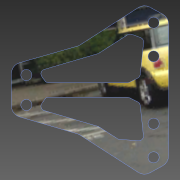
# Autodesk Inventor part: ShoulderBracket
Saved by Autodesk Inventor 2020 (Build 240168000, 168)
## iProperties
Created: 2020-04-01
Part Number: ShoulderBracket
Material: Aluminum 6061
Document SubType Name: Modeling
Designer: valer
Density: 2.7 g/cm^3
Appearance: Aluminum - Flat
Author: valer
Autodesk Inventor part; units mm, degrees
ref_plane "YZ Plane" through (0, 0, 0) normal (1, 0, 0) x (0, 1, 0)
ref_plane "XZ Plane" through (0, 0, 0) normal (0, 1, 0) x (-1, 0, 0)
ref_plane "XY Plane" through (0, 0, 0) normal (0, 0, 1) x (1, 0, 0)
sketch "Base" plane through (0, 0, 0) normal (0, 0, 1) x (1, 0, 0)
  line L0 (0, 0) -> (-82.3214, 0) construction
  line L1 (0, 0) -> (0, -41.0722)
  line L2 (-50.837, -25.008) -> (-13.8922, -48.6905)
  line L3 (-13.8922, -48.6905) -> (0, -41.0722)
  line L4 (-28.3819, -27.8847) -> (-13.9014, -28.9375)
  line L5 (-23.3971, -3.7633) -> (-16.1703, -7.3501)
  line L6 (-69.1942, -4.064) -> (-73.825, -10.6243)
  line L7 (-69.1942, -4.064) -> (-22.7911, -4.064)
  line L8 (-73.825, -10.6243) -> (-39.6875, -20.6375)
  line L9 (-16.1703, -7.3501) -> (-13.9014, -28.9375)
  line L10 (-39.6875, -20.6375) -> (-28.3819, -27.8847)
  line L11 (-88.9, 14.1014) -> (-88.9, -13.8433)
  line L12 (0, 0) -> (0, 41.0722)
  line L13 (-50.837, 25.008) -> (-13.8922, 48.6905)
  line L14 (-13.8922, 48.6905) -> (0, 41.0722)
  line L15 (-22.0332, 31.9543) -> (-13.9014, 28.9375)
  line L16 (-22.7911, 4.064) -> (-16.1703, 7.3501)
  line L17 (-69.1942, 4.064) -> (-73.825, 10.6243)
  line L18 (-69.1942, 4.064) -> (-22.7911, 4.064)
  line L19 (-73.825, 10.6243) -> (-39.6875, 20.6375)
  line L20 (-16.1703, 7.3501) -> (-13.9014, 28.9375)
  line L21 (-39.6875, 20.6375) -> (-22.0332, 31.9543)
  line L22 (-50.837, -25.008) -> (-88.9, -13.8433)
  line L23 (-50.837, 25.008) -> (-88.9, 14.1014)
  dimension "d39" = 82.3214
  dimension "d44" = 4.064
  constraints: 48 end point, 5 symmetric about line, 2 horizontal, 2 vertical, 1 parallel, 1 point on line, 2 other
  measures "d39" distance of point (0, 0) L0.end
  measures "d44" distance between parallel lines of L7 L0
extrude "Extrusion3" add sketch "Base" along normal blind 5.08
fillet "Fillet5" radius 6.35 8 edges at (-13.8922, 48.6905, 2.54) (0, 41.0722, 2.54) (-88.9, 14.1014, 2.54) (-88.9, -13.8433, 2.54) (-50.837, -25.008, 2.54) (-13.8922, -48.6905, 2.54) (0, -41.0722, 2.54) (-50.837, 25.008, 2.54)
fillet "Fillet6" radius 2.54 14 edges at (-73.825, 10.6243, 2.54) (-73.825, -10.6243, 2.54) (-69.1942, -4.064, 2.54) (-69.1942, 4.064, 2.54) (-39.6875, 20.6375, 2.54) (-22.0332, 31.9543, 2.54) (-13.9014, 28.9375, 2.54) (-16.1703, 7.3501, 2.54) (-22.7911, 4.064, 2.54) (-22.7911, -4.064, 2.54) (-16.1703, -7.3501, 2.54) (-13.9014, -28.9375, 2.54) (-28.3819, -27.8847, 2.54) (-39.6875, -20.6375, 2.54)
sketch "Sketch6" plane through (0, 0, 5.08) normal (0, 0, 1) x (1, 0, 0)
  line L0 (-106.68, 0) -> (17.78, 0) projected
  line L1 (-8.4667, 0) -> (-8.4667, -38.1) construction
  line L2 (0, -37.3123) -> (0, 37.3123) projected
  circle A0 centre (-8.4667, -19.05) radius 3.175
  circle A1 centre (-8.4667, -38.1) radius 3.175
  circle A2 centre (-80.4333, -8.4667) radius 3.175
  line L3 (-88.9, 9.3154) -> (-88.9, -9.0884) projected
  circle A3 centre (-8.4667, 19.05) radius 3.175
  circle A4 centre (-8.4667, 38.1) radius 3.175
  circle A5 centre (-80.4333, 8.4667) radius 3.175
  point P0 (0, 0)
  dimension "d49" = 8.4667
  dimension "d50" = 38.1
  dimension "d51" = 6.35
  dimension "d53" = 8.4667
  dimension "d54" = 8.4667
  constraints: 6 centre point, 3 symmetric about line, 2 end point, 2 equal radius, 1 coincident, 1 midpoint, 1 point on line, 1 vertical, 3 other
  measures "d49" distance between parallel lines of L2 L1
  measures "d50" distance of L1.start L1.end
  measures "d51" diameter of A0
  measures "d53" distance from line of L0 A2.centre
  measures "d54" distance from line of L3 A2.centre
extrude "Extrusion5" cut sketch "Sketch6" against normal blind 5.08
body "Solid2"
